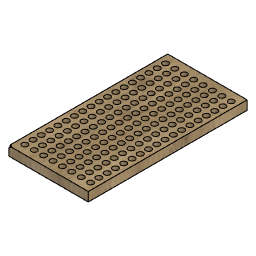
Piatto v21 (Autodesk Fusion 360 design; units mm, degrees)
Autodesk Fusion 360 part; units mm, degrees
sketch "Sketch3" plane through (0, 0, 0) normal (0, 0, 1) x (1, 0, 0)
  line L0 (175, 350) -> (-175, 350)
  line L1 (-175, 350) -> (-175, -350)
  line L2 (-175, -350) -> (175, -350)
  line L3 (175, -350) -> (175, 350)
  line L4 (175, 350) -> (-175, -350) construction
  line L5 (-175, 350) -> (175, -350) construction
  dimension "d56" = 350
  dimension "d57" = 700
  constraint perpendicular L0 L1
  constraint parallel L0 L2
  constraint parallel L1 L3
  constraint horizontal L0
  constraint coincident L4 origin
  constraint coincident L5 origin
  measures "d56" distance of L1.end L2.end
  measures "d57" distance of L0.end L1.end
extrude "Extrude1" add sketch "Sketch3" along normal blind 40 in component "Piatto"
hole "Hole1" at (-143.9599, 309.2436, 40) direction (0, 0, -1) diameter 25 end through all in component "Piatto"
pattern_linear "R-Pattern1" count 18 spacing 36.4706 along (0, -1, 0) count 8 spacing 41.4286 along (1, 0, 0) of "Hole1" in component "Piatto"
sketch "Sketch4" plane through (0, -350, 0) normal (0, -1, 0) x (1, 0, 0)
  line L0 (-175, 0) -> (175, 0)
  line L1 (175, 0) -> (175, 40)
  line L2 (175, 40) -> (-175, 40)
  line L3 (-175, 40) -> (-175, 0)
  circle A0 centre (-175, 40) radius 7.5
  dimension "d60" = 15
  constraint coincident L2.end L3.start
  measures "d60" diameter of A0
extrude "Extrude3" cut sketch "Sketch4" against normal blind 5 contours L2 L3 A0 picked at (-173.2571, 35.3272) in component "Piatto"
component "Piatto" placed x (1, 0, 0) y (0, 1, 0) z (0, 0, 1) at (0, 0, 0)
